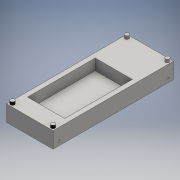
# Autodesk Inventor part: BaseBluetooth
Saved by Autodesk Inventor 2016 (Build 200138000, 138)
## iProperties
Created: 2016-04-23
Part Number: BaseBluetooth
Material: Generic
Document SubType Name: Modeling
Designer: Freddy Chang
Density: 1 g/cm^3
Appearance: Default
Author: Freddy Chang
Autodesk Inventor part; units mm, degrees
ref_plane "YZ Plane" through (0, 0, 0) normal (1, 0, 0) x (0, 1, 0)
ref_plane "XZ Plane" through (0, 0, 0) normal (0, 1, 0) x (-1, 0, 0)
ref_plane "XY Plane" through (0, 0, 0) normal (0, 0, 1) x (1, 0, 0)
sketch "Sketch1" plane through (0, 0, 0) normal (0, 0, 1) x (1, 0, 0)
  line L0 (0, 0) -> (23.2, 0)
  line L1 (23.2, 0) -> (23.2, -60)
  line L2 (23.2, -60) -> (0, -60)
  line L3 (0, -60) -> (0, 0)
  dimension "d0" = 23.2
  dimension "d1" = 60
  constraints: 8 end point, 2 parallel, 1 horizontal, 1 perpendicular
  measures "d0" distance of L1.end L2.end
  measures "d1" distance of L0.end L1.end
extrude "Extrusion1" add sketch "Sketch1" along normal blind 8
sketch "Sketch2" plane through (0, 0, 8) normal (0, 0, 1) x (1, 0, 0)
  line L0 (23.2, 0) -> (0, 0) projected
  line L1 (2.325, -3) -> (20.875, -3)
  line L2 (20.875, -3) -> (20.875, -57)
  line L3 (20.875, -57) -> (2.325, -57)
  line L4 (2.325, -57) -> (2.325, -3)
  line L5 (0, 0) -> (23.2, 0)
  line L6 (23.2, 0) -> (23.2, -60)
  line L7 (23.2, -60) -> (0, -60)
  line L8 (0, -60) -> (0, 0)
  dimension "d8" = 3
  dimension "d9" = 3
  dimension "d10" = 2.325
  dimension "d11" = 2.325
  constraints: 16 end point, 4 parallel, 2 horizontal, 2 perpendicular
  measures "d8" distance between parallel lines of L0 L1
  measures "d9" distance between parallel lines of L3 L7
  measures "d10" distance between parallel lines of L6 L2
  measures "d11" distance between parallel lines of L8 L4
extrude "Extrusion2" cut sketch "Sketch2" against normal blind 5.5 contours L1 L2 L3 L4
sketch "Sketch3" plane through (0, -60, 0) normal (-1, 0, 0) x (0, 0, 1)
  circle A0 centre (2, 57) radius 0.5
  line L0 (0, 60) -> (8, 60) projected
  line L1 (0, 60) -> (0, 0) projected
  circle A1 centre (2, 3) radius 0.5
  line L2 (0, 0) -> (8, 0) projected
  dimension "d16" = 1
  dimension "d17" = 3
  dimension "d21" = 1
  dimension "d22" = 2
  dimension "d23" = 3
  dimension "d24" = 2
  constraints: 2 centre point
  measures "d16" diameter of A0
  measures "d17" distance from line of L0 A0.centre
  measures "d21" diameter of A1
  measures "d22" distance from line of L1 A1.centre
  measures "d23" distance from line of L2 A1.centre
  measures "d24" distance from line of L1 A0.centre
extrude "Extrusion3" cut sketch "Sketch3" against normal blind 25
sketch "Sketch4" plane through (0, 0, 8) normal (0, 0, 1) x (1, 0, 0)
  line L0 (2.325, -57) -> (2.325, -3) projected
  circle A0 centre (1.5, -1.5) radius 1
  line L1 (20.875, -57) -> (2.325, -57) projected
  line L2 (20.875, -3) -> (20.875, -57) projected
  line L3 (2.325, -3) -> (20.875, -3) projected
  line L4 (20.875, -3) -> (20.875, -4.1486)
  circle A1 centre (21.7, -1.5) radius 1
  circle A2 centre (21.7, -58.5) radius 1
  circle A3 centre (1.5, -58.5) radius 1
  line L5 (0, -60) -> (23.2, -60) projected
  line L6 (23.2, -60) -> (23.2, 0) projected
  line L7 (23.2, 0) -> (0, 0) projected
  line L8 (0, 0) -> (0, -60) projected
  dimension "d27" = 2
  dimension "d29" = 2
  dimension "d31" = 2
  dimension "d32" = 2
  dimension "d34" = 1.5
  dimension "d35" = 1.5
  dimension "d36" = 1.5
  dimension "d37" = 1.5
  dimension "d38" = 1.5
  dimension "d39" = 1.5
  dimension "d40" = 1.5
  dimension "d41" = 1.5
  constraints: 4 centre point, 2 end point, 1 point on line
  measures "d27" diameter of A0
  measures "d29" diameter of A1
  measures "d31" diameter of A2
  measures "d32" diameter of A3
  measures "d34" distance from line of L5 A3.centre
  measures "d35" distance from line of L6 A2.centre
  measures "d36" distance from line of L5 A2.centre
  measures "d37" distance from line of L6 A1.centre
  measures "d38" distance from line of L7 A1.centre
  measures "d39" distance from line of L8 A3.centre
  measures "d40" distance from line of L8 A0.centre
  measures "d41" distance from line of L7 A0.centre
extrude "Extrusion4" add sketch "Sketch4" along normal blind 1.5 contours A0 | A1 | A2 | A3
sketch "Sketch6" plane through (0, 0, 2.5) normal (0, 0, 1) x (1, 0, 0)
  line L0 (2.325, -3) -> (20.875, -3) projected
  line L1 (20.875, -57) -> (2.325, -57) projected
  line L2 (2.325, -18.125) -> (20.875, -18.125)
  line L3 (20.875, -51.875) -> (2.325, -51.875)
  line L4 (2.325, -51.875) -> (2.325, -18.125)
  line L5 (23.2, -60) -> (23.2, 0) projected
  line L6 (20.875, -18.125) -> (20.875, -51.875)
  line L7 (2.325, -57) -> (2.325, -3) projected
  line L8 (2.325, -3) -> (20.875, -3)
  line L9 (20.875, -3) -> (20.875, -18.125)
  line L10 (20.875, -18.125) -> (2.325, -18.125)
  line L11 (2.325, -18.125) -> (2.325, -3)
  line L12 (2.325, -51.875) -> (20.875, -51.875)
  line L13 (20.875, -51.875) -> (20.875, -57)
  line L14 (20.875, -57) -> (2.325, -57)
  line L15 (2.325, -57) -> (2.325, -51.875)
  point P0 (0, 0)
  dimension "d46" = 15.125
  dimension "d47" = 5.125
  dimension "d49" = 20.875
  constraints: 24 end point, 5 parallel, 3 horizontal, 3 perpendicular
  measures "d46" distance between parallel lines of L0 L2
  measures "d47" distance between parallel lines of L1 L3
  measures "d49" distance between parallel lines of L5 L4
extrude "Extrusion5" add sketch "Sketch6" along normal blind 5.5 contours L0 L9 L2 L7 | L3 L13 L1 L7
body "Solid1"
